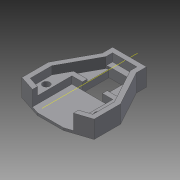
# Autodesk Inventor part: InkjetHolderV5
Saved by Autodesk Inventor 2015 (Build 190159000, 159)
## iProperties
Created: 2015-06-18
Part Number: InkjetHolderV5
Material: Generic
Document SubType Name: Modeling
Designer: Oliver
Density: 1 g/cm^3
Appearance: Default
Author: Oliver
Autodesk Inventor part; units mm, degrees
ref_plane "YZ Plane" through (0, 0, 0) normal (1, 0, 0) x (0, 1, 0)
ref_plane "XZ Plane" through (0, 0, 0) normal (0, 1, 0) x (-1, 0, 0)
ref_plane "XY Plane" through (0, 0, 0) normal (0, 0, 1) x (1, 0, 0)
sketch "Sketch1" plane through (0, 0, 0) normal (0, 0, 1) x (1, 0, 0)
  line L0 (-5, -2.5) -> (5, -2.5) construction
  line L1 (5, -2.5) -> (12.675, 0) construction
  line L2 (-5, -2.5) -> (-12.675, 0)
  line L3 (12.675, 0) -> (-12.675, 0) construction
  line L4 (12.675, 0) -> (12.675, 8.7) construction
  line L5 (-12.675, 0) -> (-12.675, 8.7)
  line L6 (-12.675, 8.7) -> (-4.75, 23.2)
  line L7 (-4.75, 23.2) -> (-4.75, 25.7)
  line L8 (-4.75, 25.7) -> (4.75, 25.7) construction
  line L9 (4.75, 25.7) -> (4.75, 23.2) construction
  line L10 (4.75, 23.2) -> (12.675, 8.7) construction
  line L11 (0, -8.56) -> (0, 31.76) projected
  line L12 (0, 25.7) -> (0, -2.5)
  circle A0 centre (-10.8, 4.25) radius 1.25
  line L13 (-10.8, 4.25) -> (0, 4.25) construction
  line L14 (-4.75, 25.7) -> (0, 25.7)
  line L15 (-5, -2.5) -> (0, -2.5)
  line L16 (-5.05, 23.2766) -> (-12.975, 8.7766)
  line L17 (-12.975, 8.7766) -> (-12.975, -0.2178)
  line L18 (-12.975, -0.2178) -> (-5.0476, -2.8)
  line L19 (-5.0476, -2.8) -> (0.3, -2.8) construction
  line L20 (0.3, -2.8) -> (0.3, 26) construction
  line L21 (0.3, 26) -> (-5.05, 26) construction
  line L22 (-5.05, 26) -> (-5.05, 23.2766)
  line L23 (0, -2.5) -> (0, -2.8)
  line L24 (0, 25.7) -> (0, 26)
  line L25 (0, -2.8) -> (-5.0476, -2.8)
  line L26 (0, 26) -> (-5.05, 26)
  point P0 (0, 0)
  point P1 (0, 0)
  dimension "d0" = 10
  dimension "d1" = 25.35
  dimension "d2" = 2.5
  dimension "d3" = 8.7
  dimension "d4" = 28.2
  dimension "d6" = 2.5
  dimension "d7" = 9.5
  dimension "d42" = 2.5
  dimension "d43" = 10.8
  dimension "d44" = 6.75
  dimension "d53" = 0.3
  constraints: 52 end point, 7 point on line, 4 equal length, 4 horizontal, 4 vertical, 3 collinear, 3 midpoint, 1 centre point, 1 coincident, 1 perpendicular, 6 other
  measures "d0" distance of L0.start L0.end
  measures "d1" distance of L1.end L2.end
  measures "d2" distance between parallel lines of L3 L0
  measures "d3" distance of L1.end L4.end
  measures "d4" distance between parallel lines of L0 L8
  measures "d6" distance of L8.end L9.end
  measures "d7" distance of L7.end L8.end
  measures "d42" diameter of A0
  measures "d43" distance of L13.start L13.end
  measures "d44" distance between parallel lines of L0 L13
  measures "d53" distance between parallel lines of L6 L16
sketch "Sketch8" plane through (0, 0, 0) normal (0, 0, 1) x (1, 0, 0)
  line L0 (-20, 30) -> (20, 30)
  line L1 (20, 30) -> (20, -10)
  line L2 (20, -10) -> (-20, -10)
  line L3 (-20, -10) -> (-20, 30)
  point P0 (0, 0)
  point P1 (0, -10)
  dimension "d45" = 40
  dimension "d46" = 10
  constraints: 8 end point, 2 parallel, 2 perpendicular, 1 horizontal, 1 midpoint, 1 vertical alignment
  measures "d45" distance of L1.end L2.end
  measures "d46" distance from line of L2 point (0, 0)
extrude "MainBlock" add sketch "Sketch8" against normal blind 7
extrude "CartridgeCutout" cut sketch "Sketch1" against normal blind 3
sketch "Sketch10" plane through (-10.8, 4.25, 0) normal (0, 0, 1) x (1, 0, 0)
  circle A0 centre (0, 0) radius 1.25 projected
  circle A1 centre (0, 0) radius 1.45
  point P0 (10.8, -4.25)
  dimension "d56" = 0.2
  constraints: 1 centre point
  measures "d56" radial gap between concentric circles of A0 A1
extrude "PinHole" cut sketch "Sketch10" against normal through all contours A0 | A1
mirror "Mirror3" about plane through (0, 26, 0) normal (-1, 0, 0) of "CartridgeCutout", "PinHole"
sketch "Sketch12" plane through (0, 0, -3) normal (0, 0, 1) x (1, 0, 0)
  circle A0 centre (10.8, 4.25) radius 1.45 projected
  circle A1 centre (-10.8, 4.25) radius 1.45 projected
  line L0 (5.05, 26) -> (-5.05, 26) projected
  line L1 (-5.05, 23.2766) -> (-5.05, 26) projected
  line L2 (-12.975, 8.7766) -> (-5.05, 23.2766) projected
  line L3 (-12.975, -0.2178) -> (-12.975, 8.7766) projected
  line L4 (-5.0476, -2.8) -> (-12.975, -0.2178) projected
  line L5 (5.0476, -2.8) -> (-5.0476, -2.8) projected
  line L6 (5.0476, -2.8) -> (12.975, -0.2178) projected
  line L7 (12.975, -0.2178) -> (12.975, 8.7766) projected
  line L8 (12.975, 8.7766) -> (5.05, 23.2766) projected
  line L9 (5.05, 23.2766) -> (5.05, 26) projected
  line L10 (-4.15, 23.6) -> (4.15, 23.6)
  line L11 (4.15, 23.6) -> (4.15, -1.4)
  line L12 (4.15, -1.4) -> (-4.15, -1.4)
  line L13 (-4.15, -1.4) -> (-4.15, 23.6)
  point P0 (0, 0)
  point P1 (0, -1.4)
  dimension "d59" = 8.3
  dimension "d60" = 25
  dimension "d61" = 1.4
  constraints: 8 end point, 2 parallel, 1 horizontal, 1 midpoint, 1 perpendicular, 1 vertical alignment
  measures "d59" distance of L11.end L12.end
  measures "d60" distance of L10.end L11.end
  measures "d61" distance from line of L12 point (0, 0)
extrude "CentreHole" cut sketch "Sketch12" against normal through all contours L10 L11 L12 L13
sketch "Sketch13" plane through (0, 0, 0) normal (0, 0, 1) x (1, 0, 0)
  line L0 (-5.05, 26) -> (5.05, 26) projected
  line L1 (5.05, 26) -> (5.05, 23.2766) projected
  line L2 (5.05, 23.2766) -> (12.975, 8.7766) projected
  line L3 (12.975, 8.7766) -> (12.975, -0.2178) projected
  line L4 (12.975, -0.2178) -> (5.0476, -2.8) projected
  line L5 (5.0476, -2.8) -> (-5.0476, -2.8) projected
  line L6 (-5.0476, -2.8) -> (-12.975, -0.2178) projected
  line L7 (-12.975, -0.2178) -> (-12.975, 8.7766) projected
  line L8 (-12.975, 8.7766) -> (-5.05, 23.2766) projected
  line L9 (-5.05, 23.2766) -> (-5.05, 26) projected
  line L10 (-20, 30) -> (20, 30) projected
  line L11 (-20, -10) -> (-20, 30) projected
  line L12 (20, -10) -> (-20, -10) projected
  line L13 (20, 30) -> (20, -10) projected
  line L14 (-14.975, 9.2875) -> (-14.975, -1.6698)
  line L15 (-14.975, -1.6698) -> (-5.3652, -4.8)
  line L16 (-5.3652, -4.8) -> (5.3652, -4.8)
  line L17 (5.3652, -4.8) -> (14.975, -1.6698)
  line L18 (14.975, -1.6698) -> (14.975, 9.2875)
  line L19 (14.975, 9.2875) -> (7.05, 23.7875)
  line L20 (7.05, 23.7875) -> (7.05, 28)
  line L21 (7.05, 28) -> (-7.05, 28)
  line L22 (-7.05, 28) -> (-7.05, 23.7875)
  line L23 (-7.05, 23.7875) -> (-14.975, 9.2875)
  point P0 (0, 0)
  dimension "d65" = 2
  constraints: 20 end point, 9 other
  measures "d65" distance between parallel lines of L7 L14
extrude "OutlineCut" cut sketch "Sketch13" against normal through all contours L10 L13 L12 L11
sketch "Sketch14" plane through (0, 0, -3) normal (0, 0, 1) x (1, 0, 0)
  line L0 (-4.15, -1.4) -> (-4.15, 23.6) projected
  line L1 (-4.15, 23.6) -> (4.15, 23.6) projected
  line L2 (4.15, 23.6) -> (4.15, -1.4) projected
  line L3 (4.15, -1.4) -> (-4.15, -1.4) construction
  circle A0 centre (10.8, 4.25) radius 1.45 construction
  circle A1 centre (-10.8, 4.25) radius 1.45 construction
  line L4 (5.05, 26) -> (-5.05, 26) projected
  line L5 (-5.05, 23.2766) -> (-5.05, 26) projected
  line L6 (-12.975, 8.7766) -> (-5.05, 23.2766) projected
  line L7 (-12.975, -0.2178) -> (-12.975, 8.7766) construction
  line L8 (-5.0476, -2.8) -> (-12.975, -0.2178) construction
  line L9 (5.0476, -2.8) -> (-5.0476, -2.8) construction
  line L10 (5.0476, -2.8) -> (12.975, -0.2178) construction
  line L11 (12.975, -0.2178) -> (12.975, 8.7766) construction
  line L12 (12.975, 8.7766) -> (5.05, 23.2766) projected
  line L13 (5.05, 23.2766) -> (5.05, 26) projected
  line L14 (-9.7922, 14.6) -> (-4.15, 14.6)
  line L15 (-12.975, 8.7766) -> (-5.05, 23.2766) projected
  line L16 (-4.15, 23.6) -> (-5.05, 23.2766)
  line L17 (0, -18) -> (0, 38) projected
  line L18 (-4.15, 23.6) -> (-4.15, 14.6)
  line L19 (-4.15, -1.4) -> (-4.15, 23.6) projected
  line L20 (-5.05, 23.2766) -> (-9.7922, 14.6)
  line L21 (-12.975, 8.7766) -> (-5.05, 23.2766) projected
  line L22 (9.7922, 14.6) -> (4.15, 14.6)
  line L23 (4.15, 23.6) -> (5.05, 23.2766)
  line L24 (4.15, 23.6) -> (4.15, 14.6)
  line L25 (5.05, 23.2766) -> (9.7922, 14.6)
  point P0 (0, 0)
  dimension "d70" = 9
  constraints: 16 end point, 2 collinear, 2 point on line, 2 symmetric about line, 1 perpendicular
  measures "d70" distance of L14.end L0.end
extrude "AlignmentGooveCut" cut sketch "Sketch14" against normal blind 1 contours L14 L6 L16 L0 | L23 L12 L22 L2
sketch "Sketch16" plane through (0, 0, 0) normal (0, 0, 1) x (1, 0, 0)
  line L0 (-8.5, 12.6) -> (8.5, 12.6)
  line L1 (8.5, 12.6) -> (8.5, -7.4)
  line L2 (8.5, -7.4) -> (-8.5, -7.4)
  line L3 (-8.5, -7.4) -> (-8.5, 12.6)
  line L4 (4.15, -1.4) -> (-4.15, -1.4) projected
  point P0 (0, 0)
  point P1 (0, -7.4)
  dimension "d73" = 17
  dimension "d74" = 20
  dimension "d75" = 14
  constraints: 8 end point, 2 parallel, 1 horizontal, 1 midpoint, 1 perpendicular, 1 vertical alignment
  measures "d73" distance of L0.start L0.end
  measures "d74" distance of L0.end L1.end
  measures "d75" distance between parallel lines of L0 L4
extrude "CircuitBoardCut" cut sketch "Sketch16" against normal blind 6
sketch "Sketch18" plane through (0, 0, -6) normal (0, 0, 1) x (1, 0, 0)
  line L0 (-4.15, 12.6) -> (-4.15, -1.4) projected
  line L1 (-4.15, -1.4) -> (4.15, -1.4) projected
  line L2 (4.15, -1.4) -> (4.15, 12.6) projected
  line L3 (-4.15, 12.6) -> (4.15, 12.6)
  line L4 (-4.15, 23.6) -> (-4.15, -1.4) projected
  point P0 (0, 0)
  constraints: 2 end point, 1 perpendicular
extrude "CircuitBoardFillIn" add sketch "Sketch18" against normal up to surface (1 mm away)
sketch "Sketch19" plane through (0, 0, 0) normal (0, 0, 1) x (1, 0, 0)
  line L0 (8.5, -1.6754) -> (8.5, -3.7789) projected
  line L1 (8.5, -3.7789) -> (14.975, -1.6698) projected
  line L2 (14.975, -1.6698) -> (14.975, 9.2875) projected
  line L3 (14.975, 9.2875) -> (7.05, 23.7875) projected
  line L4 (7.05, 23.7875) -> (7.05, 28) projected
  line L5 (-7.05, 28) -> (-7.05, 23.7875) projected
  line L6 (-7.05, 23.7875) -> (-14.975, 9.2875) projected
  line L7 (-14.975, 9.2875) -> (-14.975, -1.6698) projected
  line L8 (-14.975, -1.6698) -> (-8.5, -3.7789) projected
  line L9 (-8.5, -3.7789) -> (-8.5, -1.6754) projected
  line L10 (-8.5, -1.6754) -> (-12.975, -0.2178) projected
  line L11 (-12.975, -0.2178) -> (-12.975, 8.7766) projected
  line L12 (-12.975, 8.7766) -> (-5.05, 23.2766) projected
  line L13 (-5.05, 23.2766) -> (-5.05, 26) projected
  line L14 (-5.05, 26) -> (5.05, 26) projected
  line L15 (5.05, 26) -> (5.05, 23.2766) projected
  line L16 (5.05, 23.2766) -> (12.975, 8.7766) projected
  line L17 (12.975, 8.7766) -> (12.975, -0.2178) projected
  line L18 (12.975, -0.2178) -> (8.5, -1.6754) projected
  line L19 (7.05, 28) -> (-7.05, 28) projected
  point P0 (0, 0)
extrude "TopHeightAdjustment" add sketch "Sketch19" along normal blind 0.3
body "Solid4"
